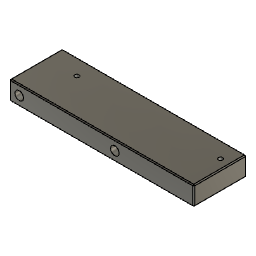
PSU Mount v1 (Autodesk Fusion 360 design; units mm, degrees)
Autodesk Fusion 360 part; units mm, degrees
sketch "Sketch1" plane through (0, 0, 0) normal (0, 0, 1) x (1, 0, 0)
  line L0 (0, 0) -> (192.5, 0)
  line L1 (192.5, 0) -> (192.5, 55)
  line L2 (192.5, 55) -> (0, 55)
  line L3 (0, 55) -> (0, 0)
  circle A0 centre (32.5, 38) radius 2.25
  circle A1 centre (182.5, 38) radius 2.25
  line L4 (32.5, 38) -> (182.5, 38) construction
  dimension "d1" = 192.5
  dimension "d2" = 55
  dimension "d3" = 150
  dimension "d4" = 4.5
  dimension "d10" = 32.5
  dimension "d11" = 17
  constraint horizontal L0
  constraint vertical L1
  constraint horizontal L2
  constraint vertical L3
  constraint coincident L0.start L3.end
  constraint coincident A0.centre L4.start
  constraint coincident A1.centre L4.end
  constraint horizontal L4
  constraint equal A0 A1
  measures "d1" distance of L0.start L0.end
  measures "d2" distance of L0.start L2.end
  measures "d3" distance of A0.centre A1.centre
  measures "d4" diameter of A0
  measures "d10" distance of L3 A0.centre
  measures "d11" distance of L2 A0.centre
extrude "Extrude1" add sketch "Sketch1" along normal blind 20
sketch "Sketch2" plane through (0, 0, 0) normal (0, 0, -1) x (1, 0, 0)
  circle A0 centre (182.5, -38) radius 2.25
  circle A1 centre (32.5, -38) radius 2.25
  line L0 (0, 0) -> (0, -55)
  line L1 (0, -55) -> (192.5, -55)
  line L2 (192.5, -55) -> (192.5, 0)
  line L3 (192.5, 0) -> (0, 0)
  circle A2 centre (32.5, -38) radius 4.5
  circle A3 centre (182.5, -38) radius 4.5
  dimension "d7" = 9
  constraint concentric A1 A2
  constraint concentric A0 A3
  constraint equal A2 A3
  measures "d7" diameter of A2
extrude "Extrude2" cut sketch "Sketch2" against normal blind 5 contours A2 | A3
sketch "Sketch3" plane through (0, 0, 0) normal (0, -1, 0) x (1, 0, 0)
  line L0 (0, 0) -> (192.5, 0)
  line L1 (192.5, 0) -> (192.5, 20)
  line L2 (192.5, 20) -> (0, 20)
  line L3 (0, 20) -> (0, 0)
  circle A0 centre (10, 10) radius 2.25
  circle A1 centre (110, 10) radius 2.25
  line L4 (10, 10) -> (110, 10) construction
  dimension "d12" = 10
  dimension "d13" = 100
  dimension "d14" = 4.5
  dimension "d15" = 10
  constraint coincident A0.centre L4.start
  constraint coincident A1.centre L4.end
  constraint parallel L0 L4
  constraint equal A0 A1
  measures "d12" distance of L0 L4
  measures "d13" distance of A0.centre A1.centre
  measures "d14" diameter of A1
  measures "d15" distance of L3 A0.centre
extrude "Extrude3" cut sketch "Sketch3" against normal through all contours A0 | A1
sketch "Sketch4" plane through (0, 0, 0) normal (0, -1, 0) x (1, 0, 0)
  circle A0 centre (10, 10) radius 2.25
  circle A1 centre (110, 10) radius 2.25
  line L0 (0, 0) -> (192.5, 0)
  line L1 (192.5, 0) -> (192.5, 20)
  line L2 (192.5, 20) -> (0, 20)
  line L3 (0, 20) -> (0, 0)
  circle A2 centre (10, 10) radius 4.5
  circle A3 centre (110, 10) radius 4.5
  dimension "d17" = 9
  constraint concentric A0 A2
  constraint concentric A1 A3
  constraint equal A2 A3
  measures "d17" diameter of A3
extrude "Extrude4" cut sketch "Sketch4" against normal blind 50 contours A2 | A3
chamfer "Chamfer1" distance 1 angle 45 12 edges at (96.25, 0, 20) (192.5, 27.5, 20) (96.25, 55, 20) (0, 27.5, 20) (0, 0, 10) (96.25, 0, 0) (192.5, 0, 10) (192.5, 27.5, 0) (192.5, 55, 10) (96.25, 55, 0) (0, 55, 10) (0, 27.5, 0)
